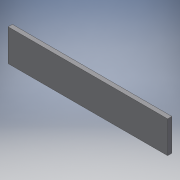
# Autodesk Inventor part: CameraBase
Saved by Autodesk Inventor 2019 (Build 230136000, 136)
## iProperties
Created: 2019-07-15
Part Number: CameraBase
Material: Generic
Document SubType Name: Modeling
Designer: aorfi
Density: 1 g/cm^3
Appearance: Default
Author: aorfi
Autodesk Inventor part; units mm, degrees
ref_plane "YZ Plane" through (0, 0, 0) normal (1, 0, 0) x (0, 1, 0)
ref_plane "XZ Plane" through (0, 0, 0) normal (0, 1, 0) x (-1, 0, 0)
ref_plane "XY Plane" through (0, 0, 0) normal (0, 0, 1) x (1, 0, 0)
sketch "Sketch1" plane through (0, 0, 0) normal (0, 0, 1) x (1, 0, 0)
  line L0 (-50, -10) -> (50, -10)
  line L1 (50, -10) -> (50, 10)
  line L2 (50, 10) -> (-50, 10)
  line L3 (-50, 10) -> (-50, -10)
  line L4 (-50, -10) -> (50, 10) construction
  line L5 (50, -10) -> (-50, 10) construction
  point P0 (0, 0)
  dimension "d2" = 100
  dimension "d3" = 20
  constraints: 12 end point, 2 midpoint, 2 parallel, 1 horizontal, 1 perpendicular
  measures "d2" distance of L0.start L0.end
  measures "d3" distance of L2.end L0.start
extrude "Extrusion1" add sketch "Sketch1" along normal mid plane 4
sketch "Sketch2" plane through (0, 0, -2) normal (0, 0, -1) x (-1, 0, 0)
  circle A0 centre (40, 2.6517) radius 1.8986
  arc A1 (46.6458, -3.9942) -> (43.9608, -1.3091) centre (45.3033, -2.6517) ccw
  line L0 (45.3033, -2.6517) -> (40, 2.6517) construction
  line L1 (40, 2.6517) -> (45.3033, 2.6517) construction
  line L2 (45.3033, 2.6517) -> (45.3033, -2.6517) construction
  circle A2 centre (40, 2.6517) radius 7.5 construction
  arc A3 (40, -2.9497) -> (40, -6.747) centre (40, -4.8483) ccw
  arc A4 (40, -6.747) -> (46.6458, -3.9942) centre (40, 2.6517) ccw
  arc A5 (40, -2.9497) -> (43.9608, -1.3091) centre (40, 2.6517) ccw
  line L3 (50, -10) -> (50, 10) construction
  line L4 (0, -15) -> (0, 15) construction
  circle A6 centre (-40, 2.6517) radius 1.8986
  arc A7 (-43.9608, -1.3091) -> (-46.6458, -3.9942) centre (-45.3033, -2.6517) ccw
  arc A8 (-40, -6.747) -> (-40, -2.9497) centre (-40, -4.8483) ccw
  arc A9 (-46.6458, -3.9942) -> (-40, -6.747) centre (-40, 2.6517) ccw
  arc A10 (-43.9608, -1.3091) -> (-40, -2.9497) centre (-40, 2.6517) ccw
  point P0 (0, 0)
  point P1 (45.3033, 0)
  point P2 (50, 0)
  dimension "d4" = 3.7973
  dimension "d5" = 3.7973
  dimension "d6" = 45
  dimension "d7" = 3.7973
  dimension "d8" = 15
  dimension "d9" = 10
  constraints: 18 point on circle, 11 centre point, 9 symmetric about line, 8 end point, 4 coincident, 2 midpoint, 2 tangent, 1 horizontal, 1 horizontal alignment, 1 perpendicular, 1 point on line, 1 vertical, 1 vertical alignment, 5 other
  measures "d4" diameter of A0
  measures "d5" diameter of A1
  measures "d6" angle of L0 L2
  measures "d7" diameter of A3
  measures "d8" diameter of A2
  measures "d9" distance from line of L0.end L3
extrude "Extrusion2" cut sketch "Sketch2" against normal through all
fillet "Fillet1" radius 2 4 edges at (-50, 10, 0) (-50, -10, 0) (50, 10, 0) (50, -10, 0)
sketch "Sketch3" plane through (0, 0, -2) normal (0, 0, -1) x (-1, 0, 0)
  line L0 (48, -10) -> (-48, -10) projected
  line L1 (7.5, -10) -> (-7.5, -10)
  line L2 (-7.5, -10) -> (-7.5, -6)
  line L3 (-7.5, -6) -> (7.5, -6)
  line L4 (7.5, -6) -> (7.5, -10)
  point P0 (0, 0)
  point P1 (0, -6)
  dimension "d13" = 15
  dimension "d14" = 4
  constraints: 8 end point, 2 parallel, 1 horizontal, 1 midpoint, 1 perpendicular, 1 point on line, 1 vertical alignment
  measures "d13" distance of L2.end L3.end
  measures "d14" distance of L1.end L2.end
extrude "Extrusion3" add sketch "Sketch3" along normal blind 15
sketch "Sketch4" plane through (-48, -10, 2) normal (0, -1, 0) x (1, 0, 0)
  line L0 (55.5, -19) -> (40.5, -19) projected
  line L1 (40.5, -4) -> (40.5, -19) projected
  point P0 (48, -2)
  point P1 (48, -11.5)
  point P2 (48, -19)
  point P3 (40.5, -11.5)
  constraints: 2 midpoint, 1 horizontal alignment, 1 vertical alignment
hole "Hole1" at (0, -10, -9.5) direction (0, 1, 0) diameter 4.496 depth 4 tip angle 118 clearance for "Flat Head Machine Screw (82)" size "#8" standard "Ansi Unified Screw Threads"
fillet "Fillet2" radius 2 4 edges at (7.5, -8, -17) (-7.5, -8, -17) (7.5, -8, -2) (-7.5, -8, -2)
equation "\"d5\" = d4"
equation "\"d7\" = d4"
body "Solid1"
